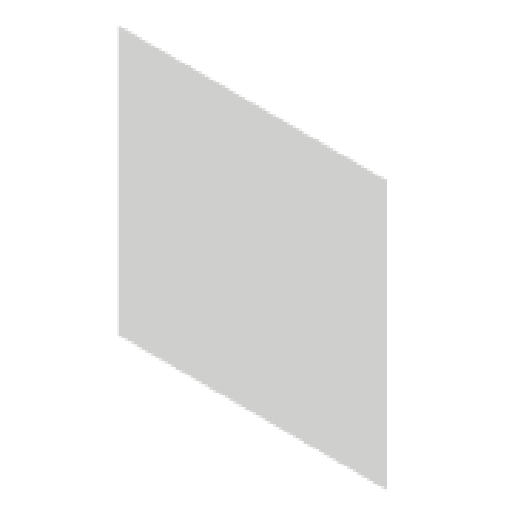
# Autodesk Inventor part: A_letter
Saved by Autodesk Inventor 2025 (Build 290162000, 162)
## iProperties
Created: 2025-01-10
Part Number: A_letter
Material: Generic
Document SubType Name: Modeling
Designer: Jan Mareš
Density: 1 g/cm^3
Appearance: Default
Author: Jan Mareš
Autodesk Inventor part; units mm, degrees
ref_plane "YZ Plane" through (0, 0, 0) normal (1, 0, 0) x (0, 1, 0)
ref_plane "XZ Plane" through (0, 0, 0) normal (0, 1, 0) x (-1, 0, 0)
ref_plane "XY Plane" through (0, 0, 0) normal (0, 0, 1) x (1, 0, 0)
sketch "Sketch1" plane through (0, 0, 0) normal (0, 0, 1) x (1, 0, 0)
  line L0 (-20, -20) -> (20, -20)
  line L1 (20, -20) -> (20, 20)
  line L2 (20, 20) -> (-20, 20)
  line L3 (-20, 20) -> (-20, -20)
  line L4 (-20, 0) -> (20, 0) construction
  line L5 (0, -28) -> (0, 28) construction
  line L6 (-28, 0) -> (28, 0) construction
  point P0 (0, 0)
  dimension "d0" = 40
  constraints: 10 end point, 3 midpoint, 2 parallel, 2 perpendicular, 1 horizontal
  measures "d0" distance of L1.end L2.end
extrude "Extrusion1" add sketch "Sketch1" along normal blind 0.6
sketch "Sketch3" plane through (0, 0, 0.6) normal (0, 0, 1) x (1, 0, 0)
  line L0 (20, -20) -> (20, 20) projected
  line L1 (20, 20) -> (-20, 20) projected
  line L2 (-20, 20) -> (-20, -20) projected
  line L3 (-20, -20) -> (20, -20) projected
  line L4 (-19.7781, -11.9695) -> (-17.1952, -4.9695) construction
  line L5 (-17.1952, -4.9695) -> (-15.1152, -4.9695) construction
  line L6 (-15.1152, -4.9695) -> (-12.5324, -11.9695) construction
  line L7 (-16.1781, -6.7695) -> (-17.0352, -9.2724) construction
  line L8 (-15.3152, -9.2724) -> (-16.1781, -6.7695) construction
  line L9 (-17.0352, -9.2724) -> (-15.3152, -9.2724) construction
  line L10 (-14.8809, -10.5581) -> (-17.4695, -10.5581) construction
  line L11 (-17.4695, -10.5581) -> (-17.9552, -11.9695) construction
  line L12 (-17.9552, -11.9695) -> (-19.7781, -11.9695) construction
  line L13 (-14.3952, -11.9695) -> (-14.8809, -10.5581) construction
  line L14 (-12.5324, -11.9695) -> (-14.3952, -11.9695) construction
  line L15 (-17.1255, -5.0695) -> (-19.6346, -11.8695)
  line L16 (-19.6346, -11.8695) -> (-18.0266, -11.8695)
  line L17 (-18.0266, -11.8695) -> (-17.5409, -10.4581)
  line L18 (-17.5409, -10.4581) -> (-14.8096, -10.4581)
  line L19 (-14.8096, -10.4581) -> (-14.3239, -11.8695)
  line L20 (-14.3239, -11.8695) -> (-12.6759, -11.8695)
  line L21 (-12.6759, -11.8695) -> (-15.1849, -5.0695)
  line L22 (-15.1849, -5.0695) -> (-17.1255, -5.0695)
  line L23 (-17.1752, -9.3724) -> (-16.1784, -6.4618)
  line L24 (-16.1784, -6.4618) -> (-15.175, -9.3724)
  line L25 (-15.175, -9.3724) -> (-17.1752, -9.3724)
  point P0 (0, 0)
  dimension "d5" = 0.1
  dimension "d6" = 0.1
  constraints: 22 end point, 9 other
  measures "d5" distance between parallel lines of L4 L15
  measures "d6" distance between parallel lines of L7 L23
extrude "Extrusion2" cut sketch "Sketch3" against normal up to next
body "Solid1"
